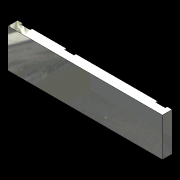
# Autodesk Inventor part: arm1_S
Saved by Autodesk Inventor 2022 (Build 260153000, 153)
## iProperties
Created: 2021-06-08
Part Number: arm1_S
Material: アルミニウム 6061
Document SubType Name: Modeling
Designer: yossy
Density: 2.7 g/cm^3
Appearance: アルミニウム - フラット
Mass: 41.04 g
Surface Area: 80.4 cm^2
Volume: 15.2 cm^3
Author: yossy
Autodesk Inventor part; units mm, degrees
ref_plane "YZ Plane" through (0, 0, 0) normal (1, 0, 0) x (0, 1, 0)
ref_plane "XZ Plane" through (0, 0, 0) normal (0, 1, 0) x (-1, 0, 0)
ref_plane "XY Plane" through (0, 0, 0) normal (0, 0, 1) x (1, 0, 0)
sketch "スケッチ1" plane through (0, 0, 0) normal (0, 0, 1) x (1, 0, 0)
  line L0 (0, 0) -> (110, 0)
  line L1 (110, 0) -> (110, 20)
  line L2 (110, 20) -> (0, 20)
  line L3 (0, 20) -> (0, 0)
  dimension "d0" = 110
  dimension "d1" = 20
  constraints: 8 end point, 2 parallel, 1 horizontal, 1 perpendicular
  measures "d0" distance of L2.end L1.end
  measures "d1" distance of L1.end L0.end
extrude "押し出し1" add sketch "スケッチ1" along normal blind 5
sketch "スケッチ2" plane through (0, 0, 0) normal (0, 0, -1) x (-1, 0, 0)
  line L0 (-110, 0) -> (-110, 20) projected
  line L1 (0, 0) -> (-110, 0) projected
  line L2 (0, 20) -> (0, 0) projected
  line L3 (-110, 20) -> (0, 20) projected
  line L4 (-2.5, 20) -> (-7.5, 20)
  line L5 (-7.5, 20) -> (-7.5, 0)
  line L6 (-7.5, 0) -> (-2.5, 0)
  line L7 (-2.5, 0) -> (-2.5, 20)
  line L8 (-107.5, 0) -> (-102.5, 0)
  line L9 (-102.5, 0) -> (-102.5, 20)
  line L10 (-102.5, 20) -> (-107.5, 20)
  line L11 (-107.5, 20) -> (-107.5, 0)
  point P0 (-107.5, 20)
  point P1 (-102.5, 0)
  dimension "d4" = 5
  dimension "d5" = 2.5
  dimension "d6" = 5
  dimension "d7" = 2.5
  constraints: 16 end point, 4 parallel, 4 point on line, 2 horizontal, 2 perpendicular
  measures "d4" distance of L6.end L5.end
  measures "d5" distance between parallel lines of L2 L7
  measures "d6" distance of L10.end L9.end
  measures "d7" distance between parallel lines of L0 L11
extrude "押し出し2" cut sketch "スケッチ2" against normal blind 1 contours L11 L3 L9 L1 | L5 L3 L7 L1
sketch "スケッチ3" plane through (0, 0, 5) normal (0, -1, 0) x (1, 0, 0)
  line L0 (30.22, -4) -> (25.22, -4) projected
  line L1 (25.22, -4) -> (25.22, -356) projected
  line L2 (25.22, -356) -> (30.22, -356) projected
  line L3 (30.22, -356) -> (30.22, -4) projected
extrude "押し出し3" cut sketch "スケッチ3" against normal through all
